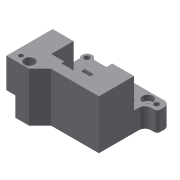
# Autodesk Inventor part: 00_Adapter_Lens_PCB_XY_Translator
Saved by Autodesk Inventor 2019 (Build 230136000, 136)
## iProperties
Created: 2018-09-10
Part Number: 00_Adapter_Lens_PCB_XY_Translator
Material: Generisch
Document SubType Name: Modeling
Designer: Henry John
Density: 1 g/cm^3
Appearance: Vorgabe
Author: Henry John
Autodesk Inventor part; units mm, degrees
ref_plane "YZ Plane" through (0, 0, 0) normal (1, 0, 0) x (0, 1, 0)
ref_plane "XZ Plane" through (0, 0, 0) normal (0, 1, 0) x (-1, 0, 0)
sketch "Skizze1" plane through (0, 0, 0) normal (0, 0, 1) x (1, 0, 0)
  line L0 (14.1792, -15.989) -> (14.1792, 19.011)
  line L1 (14.1792, 19.011) -> (-11.8208, 19.011)
  line L2 (-11.8208, 19.011) -> (-11.8208, -15.989)
  line L3 (-11.8208, -15.989) -> (14.1792, -15.989)
  line L4 (14.1792, -15.989) -> (-11.8208, 19.011) construction
  line L5 (14.1792, 19.011) -> (-11.8208, -15.989) construction
  line L6 (3.4292, 11.636) -> (-6.0708, 11.636) construction
  line L7 (3.4292, 4.386) -> (3.4292, 11.636) construction
  line L8 (-6.0708, 3.091) -> (3.4292, 3.091) construction
  line L9 (-6.0708, 11.636) -> (-6.0708, 4.386) construction
  line L10 (3.4292, 11.636) -> (-6.0708, 4.386) construction
  line L11 (3.4292, 4.386) -> (-6.0708, 11.636) construction
  point P0 (0, 0)
  point P1 (1.1792, 1.511)
  point P2 (1.1792, 1.511)
  point P3 (-1.3208, 8.011)
  point P4 (-1.3208, 8.011)
  point P5 (1.1792, 1.511)
  point P6 (-1.3208, 8.011)
  dimension "d0" = 26
  dimension "d1" = 35
  dimension "d2" = 11
  dimension "d3" = 2.5
  constraints: 16 end point, 6 midpoint, 2 parallel, 1 coincident, 1 perpendicular, 1 vertical
  measures "d0" distance of L1.end L0.end
  measures "d1" distance of L1.end L2.end
  measures "d2" distance from line of L1 point (-1.321, 8.011)
  measures "d3" horizontal distance of point (-1.321, 8.011) point (1.179, 1.511)
sketch "Skizze2" plane through (0, 0, 0) normal (0, 0, 1) x (1, 0, 0)
  line L0 (-3.4208, 2.386) -> (-7.8208, 2.386) projected
  line L1 (-7.8208, 2.386) -> (-7.8208, 13.636) projected
  line L2 (-7.8208, 13.636) -> (-3.4208, 13.636) projected
  line L3 (5.1792, 2.386) -> (0.7792, 2.386) projected
  line L4 (5.1792, 13.636) -> (5.1792, 2.386) projected
  line L5 (0.7792, 13.636) -> (5.1792, 13.636) projected
  circle A0 centre (-9.3002, -3.4434) radius 1.575 construction
  circle A1 centre (11.3792, 15.486) radius 1.575 construction
  circle A2 centre (-9.3002, -3.4434) radius 0.7 construction
  circle A3 centre (-10.7708, 17.311) radius 0.7 construction
  circle A4 centre (11.3792, 15.486) radius 0.7 construction
  line L6 (-3.4208, 13.636) -> (-3.4208, 14.661) projected
  line L7 (-3.4208, 14.661) -> (0.7792, 14.661) projected
  line L8 (0.7792, 1.361) -> (-3.4208, 1.361) projected
  line L9 (-3.4208, 1.361) -> (-3.4208, 2.386) projected
  line L10 (0.7792, 2.386) -> (0.7792, 1.361) projected
  line L11 (0.7792, 14.661) -> (0.7792, 13.636) projected
  line L12 (-12.2708, -7.964) -> (-12.2708, 12.036) construction
  line L13 (14.5292, 17.861) -> (-9.295, 17.861) construction
  arc A5 (16.5292, 15.861) -> (14.5292, 17.861) centre (14.5292, 15.861) ccw projected
  line L14 (16.5292, 15.861) -> (16.5292, 14.486) projected
  arc A6 (15.5292, 13.486) -> (16.5292, 14.486) centre (15.5292, 14.486) ccw projected
  line L15 (15.5292, 13.486) -> (14.4292, 13.486) projected
  arc A7 (14.4292, 13.486) -> (12.4292, 11.486) centre (14.4292, 11.486) ccw projected
  line L16 (12.4292, 11.486) -> (12.4292, -1.914) projected
  line L17 (-3.5708, -1.914) -> (12.4292, -1.914) projected
  line L18 (-8.1002, -6.4434) -> (-3.5708, -1.914) projected
  arc A8 (-10.7708, 18.886) -> (-9.295, 17.861) centre (-10.7708, 17.311) ccw construction
  line L19 (-8.1002, -7.4434) -> (-8.1002, -6.4434) construction
  circle A9 centre (-9.3002, -7.4434) radius 0.75 construction
  circle A10 centre (-9.3002, -7.4434) radius 1.2 construction
  line L20 (-10.8208, -6.614) -> (-11.8208, -5.614) construction
  line L21 (-11.8208, -5.614) -> (-11.8208, 16.0059)
  line L22 (-11.8208, -5.614) -> (-10.4976, -6.9373)
  arc A11 (-8.1002, -6.9434) -> (-8.2864, -6.6296) centre (-9.3002, -7.4434) ccw construction
  line L23 (-8.1002, -6.9434) -> (-8.1002, -6.4434) construction
  circle A12 centre (-9.3002, -3.4434) radius 1.675
  circle A13 centre (11.3792, 15.486) radius 1.675
  line L24 (14.5292, 17.861) -> (-9.1887, 17.861)
  arc A14 (-11.8208, 16.0059) -> (-9.1887, 17.861) centre (-10.7708, 17.311) ccw
  circle A15 centre (14.3792, 15.486) radius 0.75 construction
  circle A16 centre (14.3792, 15.486) radius 0.85
  line L25 (-8.1002, -6.4434) -> (-8.2864, -6.6296) construction
  arc A17 (-8.2864, -6.6296) -> (-10.4976, -6.9373) centre (-9.3002, -7.4434) ccw construction
  line L26 (-11.8208, -5.614) -> (-7.2708, -5.614)
  point P0 (0, 0)
  dimension "d4" = 0.1
  dimension "d5" = 0.1
  dimension "d6" = 0.1
  dimension "d7" = 0.1
  dimension "d10" = 0.1
  constraints: 12 end point, 6 centre point, 6 point on circle, 5 coincident, 3 point on line, 2 collinear, 1 horizontal, 1 vertical
  measures "d4" radial gap between concentric circles of A10 A11
  measures "d5" radial gap between concentric circles of A0 A12
  measures "d6" radial gap between concentric circles of A1 A13
  measures "d7" radial gap between concentric circles of A8 A14
  measures "d10" radial gap between concentric circles of A15 A16
extrude "Extrusion1" add sketch "Skizze2" along normal blind 2.5
sketch "Skizze3" plane through (0, 0, 2.5) normal (0, 0, 1) x (1, 0, 0)
  circle A0 centre (11.3792, 15.486) radius 1.675 construction
  circle A1 centre (-9.3002, -3.4434) radius 1.675 construction
  circle A2 centre (14.3792, 15.486) radius 0.85 projected
  arc A3 (16.5292, 15.861) -> (14.5292, 17.861) centre (14.5292, 15.861) ccw projected
  line L0 (14.5292, 17.861) -> (-9.1887, 17.861) projected
  arc A4 (-11.8208, 16.0059) -> (-9.1887, 17.861) centre (-10.7708, 17.311) ccw construction
  line L1 (-11.8208, 16.0059) -> (-11.8208, -5.614) projected
  line L2 (-7.2708, -5.614) -> (-3.5708, -1.914) projected
  line L3 (-3.5708, -1.914) -> (12.4292, -1.914) projected
  line L4 (12.4292, -1.914) -> (12.4292, 11.486) projected
  arc A5 (14.4292, 13.486) -> (12.4292, 11.486) centre (14.4292, 11.486) ccw projected
  line L5 (14.4292, 13.486) -> (15.5292, 13.486) projected
  arc A6 (15.5292, 13.486) -> (16.5292, 14.486) centre (15.5292, 14.486) ccw projected
  line L6 (16.5292, 14.486) -> (16.5292, 15.861) projected
  circle A7 centre (11.3792, 15.486) radius 0.7 construction
  circle A8 centre (-9.3002, -3.4434) radius 0.7 construction
  circle A9 centre (-9.3002, -7.4434) radius 0.75 construction
  circle A10 centre (-9.3002, -7.4434) radius 0.85
  line L7 (-7.2708, -5.614) -> (-3.5708, -1.914) projected
  arc A11 (-10.3338, -7.0065) -> (-8.2864, -7.9246) centre (-9.3002, -7.4434) ccw
  arc A12 (-9.1887, 17.861) -> (-11.8208, 16.0059) centre (-10.7708, 17.311) ccw
  circle A13 centre (-10.7708, 17.311) radius 0.7 construction
  circle A14 centre (-10.7708, 17.311) radius 0.9
  circle A15 centre (11.3792, 15.486) radius 0.9
  circle A16 centre (-9.3002, -3.4434) radius 0.9
  line L8 (-11.8208, -5.614) -> (-7.2708, -5.614) projected
  line L9 (-7.8208, 2.386) -> (-7.8208, 13.636) projected
  line L10 (-7.8208, 13.636) -> (-3.4208, 13.636) projected
  line L11 (-3.4208, 13.636) -> (-3.4208, 14.661) projected
  line L12 (-3.4208, 14.661) -> (0.7792, 14.661) projected
  line L13 (0.7792, 14.661) -> (0.7792, 13.636) projected
  line L14 (0.7792, 13.636) -> (5.1792, 13.636) projected
  line L15 (5.1792, 13.636) -> (5.1792, 2.386) projected
  line L16 (5.1792, 2.386) -> (0.7792, 2.386) projected
  line L17 (0.7792, 2.386) -> (0.7792, 1.361) projected
  line L18 (0.7792, 1.361) -> (-3.4208, 1.361) projected
  line L19 (-3.4208, 1.361) -> (-3.4208, 2.386) projected
  line L20 (-3.4208, 2.386) -> (-7.8208, 2.386) projected
  circle A17 centre (11.3792, 15.486) radius 1.675 projected
  circle A18 centre (-9.3002, -3.4434) radius 1.675 projected
  circle A19 centre (14.3792, 15.486) radius 0.85 projected
  arc A20 (16.5292, 15.861) -> (14.5292, 17.861) centre (14.5292, 15.861) ccw projected
  line L21 (14.5292, 17.861) -> (-9.1887, 17.861) projected
  arc A21 (-11.8208, 16.0059) -> (-9.1887, 17.861) centre (-10.7708, 17.311) ccw projected
  line L22 (-11.8208, 16.0059) -> (-11.8208, -5.614) projected
  line L23 (-11.8208, -5.614) -> (-7.2708, -5.614) projected
  line L24 (-7.2708, -5.614) -> (-3.5708, -1.914) projected
  line L25 (-3.5708, -1.914) -> (12.4292, -1.914) projected
  line L26 (12.4292, -1.914) -> (12.4292, 11.486) projected
  arc A22 (14.4292, 13.486) -> (12.4292, 11.486) centre (14.4292, 11.486) ccw projected
  line L27 (14.4292, 13.486) -> (15.5292, 13.486) projected
  arc A23 (15.5292, 13.486) -> (16.5292, 14.486) centre (15.5292, 14.486) ccw projected
  line L28 (16.5292, 14.486) -> (16.5292, 15.861) projected
  point P0 (0, 0)
  dimension "d11" = 0.1
  dimension "d13" = 1.8
  dimension "d14" = 1.8
  dimension "d15" = 1.8
  constraints: 6 centre point, 6 coincident, 4 point on circle, 1 other
  measures "d11" radial gap between concentric circles of A9 A10
  measures "d13" diameter of A14
  measures "d14" diameter of A15
  measures "d15" diameter of A16
ref_plane "Arbeitsebene1" through (-9.7716, -9.2098, 6) normal (0, 0, 1) x (1, 0, 0)
extrude "Extrusion2" add sketch "Skizze3" along normal blind 4 contours L6 A6 L5 A5 L4 L3 L2 L8 L1 A21 L0 A3 | A21 A12 | A17 | A18
sketch "Skizze4" plane through (-9.1887, 16.566, 6.5) normal (0, 0, 1) x (1, 0, 0)
  circle A0 centre (-0.1115, -20.0094) radius 0.7 construction
  circle A1 centre (-1.5821, 0.745) radius 0.7 construction
  circle A2 centre (20.5679, -1.08) radius 0.7 construction
  point P0 (9.1887, -16.566)
hole "Bohrung1" at (-9.3002, -3.4434, 6.5) at (11.3792, 15.486, 6.5) direction (0, 0, -1) diameter 1.8 end through all counterbore diameter 3.5 counterbore depth 1.8 clearance for "Inbusschraube ISO 4762" size "M1.6" standard "ISO"
sketch "Sketch12" plane through (0, 0, 6.5) normal (0, 0, 1) x (1, 0, 0)
  circle A0 centre (-9.3002, -3.4434) radius 1.75 projected
  circle A1 centre (11.3792, 15.486) radius 1.75 projected
  line L0 (-7.8208, 13.636) -> (-3.4208, 13.636) projected
  line L1 (-3.4208, 13.636) -> (-3.4208, 14.661) projected
  line L2 (-3.4208, 14.661) -> (0.7792, 14.661) projected
  line L3 (0.7792, 14.661) -> (0.7792, 13.636) projected
  line L4 (0.7792, 13.636) -> (5.1792, 13.636) projected
  line L5 (5.1792, 13.636) -> (5.1792, 2.386) projected
  line L6 (5.1792, 2.386) -> (0.7792, 2.386) projected
  line L7 (0.7792, 2.386) -> (0.7792, 1.361) projected
  line L8 (0.7792, 1.361) -> (-3.4208, 1.361) projected
  line L9 (-3.4208, 1.361) -> (-3.4208, 2.386) projected
  line L10 (-3.4208, 2.386) -> (-7.8208, 2.386) projected
  line L11 (-7.8208, 2.386) -> (-7.8208, 13.636) projected
  circle A2 centre (14.3792, 15.486) radius 0.85 projected
  circle A3 centre (-10.7708, 17.311) radius 0.9 projected
  arc A4 (16.5292, 15.861) -> (14.5292, 17.861) centre (14.5292, 15.861) ccw projected
  line L12 (14.5292, 17.861) -> (-9.1887, 17.861) projected
  arc A5 (-9.1887, 17.861) -> (-11.8208, 16.0059) centre (-10.7708, 17.311) ccw projected
  line L13 (-11.8208, 16.0059) -> (-11.8208, -5.614) projected
  line L14 (-11.8208, -5.614) -> (-7.2708, -5.614) projected
  line L15 (-7.2708, -5.614) -> (-3.5708, -1.914) projected
  line L16 (-3.5708, -1.914) -> (12.4292, -1.914) projected
  line L17 (12.4292, -1.914) -> (12.4292, 11.486) projected
  arc A6 (14.4292, 13.486) -> (12.4292, 11.486) centre (14.4292, 11.486) ccw projected
  line L18 (14.4292, 13.486) -> (15.5292, 13.486) projected
  arc A7 (15.5292, 13.486) -> (16.5292, 14.486) centre (15.5292, 14.486) ccw projected
  line L19 (16.5292, 14.486) -> (16.5292, 15.861) projected
  line L20 (6.6092, 13.3531) -> (-8.8908, 13.3531) construction
  line L21 (-8.8908, 13.3531) -> (-8.8908, -0.1469) construction
  line L22 (-8.8908, -0.1469) -> (6.6092, -0.1469) construction
  line L23 (6.6092, -0.1469) -> (6.6092, 13.3531) construction
  circle A8 centre (-18.8908, 17.3531) radius 1 construction
  circle A9 centre (-12.3908, -3.1469) radius 1 construction
  circle A10 centre (9.1092, 12.3531) radius 1 construction
  arc A11 (-16.7463, 18.6788) -> (-17.7463, 19.6788) centre (-17.7463, 18.6788) ccw construction
  line L24 (-16.7463, 18.6788) -> (-16.7463, 15.9412) construction
  arc A12 (-16.7463, 15.9412) -> (-15.7463, 14.9412) centre (-15.7463, 15.9412) ccw construction
  line L25 (-15.7463, 14.9412) -> (10.3438, 14.9412) construction
  arc A13 (11.3438, 13.9412) -> (10.3438, 14.9412) centre (10.3438, 13.9412) ccw construction
  line L26 (11.3438, 13.9412) -> (11.3438, 11.3759) construction
  arc A14 (10.3438, 10.3759) -> (11.3438, 11.3759) centre (10.3438, 11.3759) ccw construction
  line L27 (10.3438, 10.3759) -> (10.1092, 10.3759) construction
  arc A15 (10.1092, 10.3759) -> (9.1092, 9.3759) centre (10.1092, 9.3759) ccw construction
  line L28 (9.1092, 9.3759) -> (9.1092, -2.1588) construction
  line L29 (9.1092, -2.1588) -> (-9.3631, -2.1588) construction
  arc A16 (-9.3631, -2.1588) -> (-10.3631, -3.1588) centre (-9.3631, -3.1588) ccw construction
  line L30 (-10.3631, -3.1588) -> (-10.3631, -5.0212) construction
  arc A17 (-11.3631, -6.0212) -> (-10.3631, -5.0212) centre (-11.3631, -5.0212) ccw construction
  line L31 (-11.3631, -6.0212) -> (-21.6562, -6.0212) construction
  line L32 (-21.6562, -6.0212) -> (-21.6562, 19.6788) construction
  line L33 (-21.6562, 19.6788) -> (-17.7463, 19.6788) construction
  line L34 (-7.2708, -5.614) -> (-11.8208, -5.614) construction
  line L35 (-11.8208, -5.614) -> (-14.8208, -5.614) construction
  line L36 (-14.8208, -5.614) -> (-14.8208, 15.9412) construction
  line L37 (-14.8208, 15.9412) -> (-11.8208, 15.9412) construction
  line L38 (-11.8208, 15.9412) -> (-11.8208, -5.614) construction
  line L39 (-11.8208, -5.614) -> (-14.8208, -5.614)
  line L40 (-14.8208, -5.614) -> (-14.8208, 15.9412)
  line L41 (-14.8208, 15.9412) -> (-11.8208, 15.9412)
  line L42 (-11.8208, 15.9412) -> (-11.8208, -5.614)
  point P0 (0, 0)
  dimension "d49" = 3
  constraints: 16 end point, 4 parallel, 2 horizontal, 2 perpendicular
  measures "d49" distance of L36.end L37.end
extrude "Extrusion9" add sketch "Sketch12" along normal blind 10
sketch "Sketch13" plane through (0, 0, 16.5) normal (0, 0, 1) x (1, 0, 0)
  line L0 (-5.5708, 25.836) -> (-16.7708, 25.836) construction
  arc A0 (-16.7463, 18.6788) -> (-17.7463, 19.6788) centre (-17.7463, 18.6788) ccw construction
  line L1 (-17.7463, 19.6788) -> (-21.6562, 19.6788) construction
  line L2 (-21.6562, 19.6788) -> (-21.6562, -6.0212) construction
  line L3 (-21.6562, -6.0212) -> (-11.3631, -6.0212) construction
  arc A1 (-11.3631, -6.0212) -> (-10.3631, -5.0212) centre (-11.3631, -5.0212) ccw construction
  line L4 (-10.3631, -5.0212) -> (-10.3631, -3.1588) construction
  arc A2 (-9.3631, -2.1588) -> (-10.3631, -3.1588) centre (-9.3631, -3.1588) ccw construction
  line L5 (-9.3631, -2.1588) -> (9.1092, -2.1588) construction
  line L6 (9.1092, -2.1588) -> (9.1092, 9.3759) construction
  arc A3 (10.1092, 10.3759) -> (9.1092, 9.3759) centre (10.1092, 9.3759) ccw construction
  line L7 (10.1092, 10.3759) -> (10.3438, 10.3759) construction
  arc A4 (10.3438, 10.3759) -> (11.3438, 11.3759) centre (10.3438, 11.3759) ccw construction
  line L8 (11.3438, 11.3759) -> (11.3438, 13.9412) construction
  arc A5 (11.3438, 13.9412) -> (10.3438, 14.9412) centre (10.3438, 13.9412) ccw construction
  line L9 (10.3438, 14.9412) -> (-15.7463, 14.9412) construction
  arc A6 (-16.7463, 15.9412) -> (-15.7463, 14.9412) centre (-15.7463, 15.9412) ccw construction
  line L10 (-16.7463, 15.9412) -> (-16.7463, 18.6788) construction
  line L11 (-8.8908, 13.3531) -> (6.6092, 13.3531) construction
  line L12 (6.6092, 13.3531) -> (6.6092, -0.1469) construction
  line L13 (6.6092, -0.1469) -> (-8.8908, -0.1469) construction
  line L14 (-8.8908, -0.1469) -> (-8.8908, 13.3531) construction
  circle A7 centre (-18.8908, 17.3531) radius 1 construction
  circle A8 centre (-12.3908, -3.1469) radius 1 construction
  circle A9 centre (9.1092, 12.3531) radius 1 construction
  point P0 (0, 0)
hole "Hole2" at (-12.3908, -3.1469, 16.5) at (9.1092, 12.3531, 16.5) direction (0, 0, -1) diameter 1.5 end through all
sketch "Sketch14" plane through (-14.8208, -5.614, 6.5) normal (-1, 0, 0) x (0, 0, 1)
  line L0 (0, 21.5553) -> (0, 2.9546) projected
  line L1 (19.819, 28.4609) -> (0, 28.4609)
  line L2 (0, 28.4609) -> (0, 15.475)
  line L3 (0, 15.475) -> (19.819, 15.475)
  line L4 (19.819, 15.475) -> (19.819, 28.4609)
  point P0 (-6.5, 5.614)
  constraints: 8 end point, 2 parallel, 1 horizontal, 1 perpendicular, 1 point on line
extrude "Extrusion10" cut sketch "Sketch14" against normal through all
